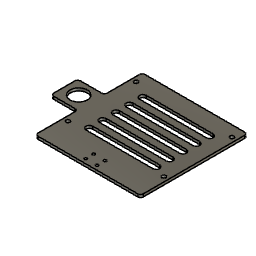
mount v1 (Autodesk Fusion 360 design; units mm, degrees)
Autodesk Fusion 360 part; units mm, degrees
sketch "Sketch1" plane through (0, 0, 0) normal (0, 0, 1) x (1, 0, 0)
  line L0 (-78.5381, -2.5381) -> (-78.5381, 7.765)
  line L1 (-76.5381, 58.0111) -> (-1.7619, 58.0111)
  line L2 (0.2381, 56.0111) -> (0.2381, -2.5381)
  circle A0 centre (-3.3, -1) radius 1.5
  circle A1 centre (-3.3, 50) radius 1.5
  circle A2 centre (-75, 50) radius 1.5
  circle A3 centre (-75, -1) radius 1.5
  line L3 (-62.5, 45) -> (-12.5, 45)
  line L4 (-12.5, 40) -> (-62.5, 40)
  line L5 (-62.5, 35) -> (-12.5, 35)
  line L6 (-12.5, 30) -> (-62.5, 30)
  line L7 (-62.5, 25) -> (-12.5, 25)
  line L8 (-12.5, 20) -> (-62.5, 20)
  line L9 (-62.5, 15) -> (-12.5, 15)
  line L10 (-12.5, 10) -> (-62.5, 10)
  line L11 (-62.5, 5) -> (-12.5, 5)
  line L12 (-12.5, 0) -> (-62.5, 0)
  arc A4 (-62.5, 45) -> (-65, 42.5) centre (-62.5, 42.5) ccw
  arc A5 (-65, 42.5) -> (-62.5, 40) centre (-62.5, 42.5) ccw
  arc A6 (-10, 42.5) -> (-12.5, 45) centre (-12.5, 42.5) ccw
  arc A7 (-12.5, 40) -> (-10, 42.5) centre (-12.5, 42.5) ccw
  arc A8 (-62.5, 35) -> (-65, 32.5) centre (-62.5, 32.5) ccw
  arc A9 (-65, 32.5) -> (-62.5, 30) centre (-62.5, 32.5) ccw
  arc A10 (-10, 32.5) -> (-12.5, 35) centre (-12.5, 32.5) ccw
  arc A11 (-12.5, 30) -> (-10, 32.5) centre (-12.5, 32.5) ccw
  arc A12 (-10, 22.5) -> (-12.5, 25) centre (-12.5, 22.5) ccw
  arc A13 (-12.5, 20) -> (-10, 22.5) centre (-12.5, 22.5) ccw
  arc A14 (-62.5, 25) -> (-65, 22.5) centre (-62.5, 22.5) ccw
  arc A15 (-65, 22.5) -> (-62.5, 20) centre (-62.5, 22.5) ccw
  arc A16 (-62.5, 15) -> (-65, 12.5) centre (-62.5, 12.5) ccw
  arc A17 (-65, 12.5) -> (-62.5, 10) centre (-62.5, 12.5) ccw
  arc A18 (-10, 12.5) -> (-12.5, 15) centre (-12.5, 12.5) ccw
  arc A19 (-12.5, 10) -> (-10, 12.5) centre (-12.5, 12.5) ccw
  arc A20 (-10, 2.5) -> (-12.5, 5) centre (-12.5, 2.5) ccw
  arc A21 (-12.5, 0) -> (-10, 2.5) centre (-12.5, 2.5) ccw
  arc A22 (-62.5, 5) -> (-65, 2.5) centre (-62.5, 2.5) ccw
  arc A23 (-65, 2.5) -> (-62.5, 0) centre (-62.5, 2.5) ccw
  line L13 (-80.5381, 29.765) -> (-96.5381, 29.765)
  line L14 (-98.5381, 27.765) -> (-98.5381, 11.765)
  line L15 (-96.5381, 9.765) -> (-80.5381, 9.765)
  circle A24 centre (-88, 20) radius 6.5
  arc A25 (-76.5381, 58.0111) -> (-78.5381, 56.0111) centre (-76.5381, 56.0111) ccw
  arc A26 (0.2381, 56.0111) -> (-1.7619, 58.0111) centre (-1.7619, 56.0111) ccw
  arc A27 (-78.5381, 7.765) -> (-80.5381, 9.765) centre (-80.5381, 7.765) ccw
  arc A28 (-96.5381, 29.765) -> (-98.5381, 27.765) centre (-96.5381, 27.765) ccw
  arc A29 (-98.5381, 11.765) -> (-96.5381, 9.765) centre (-96.5381, 11.765) ccw
  line L16 (-78.5381, 56.0111) -> (-78.5381, 31.765)
  arc A30 (-80.5381, 29.765) -> (-78.5381, 31.765) centre (-80.5381, 31.765) ccw
  line L17 (0.2381, -2.5381) -> (0.2381, -19.9889)
  line L18 (-1.7619, -21.9889) -> (-76.5381, -21.9889)
  line L19 (-78.5381, -19.9889) -> (-78.5381, -2.5381)
  arc A31 (-78.5381, -19.9889) -> (-76.5381, -21.9889) centre (-76.5381, -19.9889) ccw
  arc A32 (-1.7619, -21.9889) -> (0.2381, -19.9889) centre (-1.7619, -19.9889) ccw
  circle A33 centre (-44.1028, -12.7273) radius 1
  circle A34 centre (-35.6028, -12.7273) radius 1
  circle A35 centre (-35.6028, -18.7273) radius 1
  circle A36 centre (-44.1028, -18.7273) radius 1
  point P0 (-98.5381, 29.765)
  dimension "d1" = 71.7
  dimension "d2" = 51
  dimension "d4" = 3
  dimension "d5" = 3
  dimension "d6" = 3
  dimension "d7" = 3
  dimension "d8" = 2.5
  dimension "d9" = 2.5
  dimension "d18" = 13
  dimension "d21" = 2
  dimension "d22" = 2
  dimension "d25" = 2
  dimension "d28" = 80
  dimension "d37" = 8.5
  dimension "d38" = 6
  dimension "d39" = 2
  dimension "d40" = 2
  dimension "d41" = 2
  dimension "d42" = 2
  constraint horizontal L3
  constraint horizontal L4
  constraint horizontal L5
  constraint horizontal L6
  constraint horizontal L7
  constraint horizontal L8
  constraint horizontal L9
  constraint horizontal L10
  constraint horizontal L11
  constraint horizontal L12
  constraint tangent L3 A4
  constraint tangent L4 A5
  constraint equal A4 A5
  constraint coincident A4.end A5.start
  constraint tangent L3 A6
  constraint equal A4 A6
  constraint tangent L4 A7
  constraint equal A4 A7
  constraint coincident A6.start A7.end
  constraint tangent L5 A8
  constraint equal A4 A8
  constraint tangent L6 A9
  constraint equal A4 A9
  constraint coincident A8.end A9.start
  constraint tangent L5 A10
  constraint equal A4 A10
  constraint tangent L6 A11
  constraint equal A4 A11
  constraint coincident A10.start A11.end
  constraint tangent L7 A12
  constraint equal A4 A12
  constraint tangent L8 A13
  constraint equal A4 A13
  constraint coincident A12.start A13.end
  constraint tangent L7 A14
  constraint equal A4 A14
  constraint tangent L8 A15
  constraint equal A4 A15
  constraint coincident A14.end A15.start
  constraint tangent L9 A16
  constraint equal A4 A16
  constraint tangent L10 A17
  constraint equal A4 A17
  constraint coincident A16.end A17.start
  constraint tangent L9 A18
  constraint equal A4 A18
  constraint tangent L10 A19
  constraint equal A4 A19
  constraint coincident A18.start A19.end
  constraint tangent L11 A20
  constraint equal A4 A20
  constraint tangent L12 A21
  constraint equal A4 A21
  constraint coincident A20.start A21.end
  constraint tangent L11 A22
  constraint equal A4 A22
  constraint tangent L12 A23
  constraint coincident A22.end A23.start
  constraint horizontal L13
  constraint vertical L14
  constraint horizontal L15
  constraint tangent L1 A25
  constraint tangent L0 A25
  constraint tangent L1 A26
  constraint tangent L2 A26
  constraint equal A25 A26
  constraint coincident L0 A25.end
  constraint tangent L15 A27
  constraint tangent L0 A27
  constraint equal A25 A27
  constraint coincident P0 L13
  constraint coincident P0 L14
  constraint tangent L13 A28
  constraint tangent L14 A28
  constraint equal A25 A28
  constraint tangent L14 A29
  constraint tangent L15 A29
  constraint equal A25 A29
  constraint tangent L16 A30
  constraint tangent L13 A30
  constraint vertical L17
  constraint horizontal L18
  constraint vertical L19
  constraint tangent L19 A31
  constraint tangent L18 A31
  constraint tangent L17 A32
  constraint tangent L18 A32
  constraint equal A31 A32
  measures "d1" distance of A1.centre A2.centre
  measures "d2" distance of A2.centre A3.centre
  measures "d4" diameter of A0
  measures "d5" diameter of A1
  measures "d6" diameter of A2
  measures "d7" diameter of A3
  measures "d8" radius of A4
  measures "d9" radius of A23
  measures "d18" diameter of A24
  measures "d21" radius of A25
  measures "d22" radius of A30
  measures "d25" radius of A31
  measures "d28" distance of L1 L18
  measures "d37" distance of A35.centre A36.centre
  measures "d38" distance of A33.centre A36.centre
  measures "d39" diameter of A33
  measures "d40" diameter of A34
  measures "d41" diameter of A35
  measures "d42" diameter of A36
extrude "Extrude4" add sketch "Sketch1" along normal blind 2
